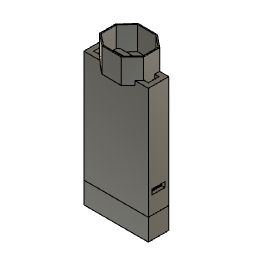
CasePCB v2 (Autodesk Fusion 360 design; units mm, degrees)
Autodesk Fusion 360 part; units mm, degrees
sketch "Schizzo1" plane through (0, 0, 0) normal (0, 0, 1) x (1, 0, 0)
  line L0 (-19.736, -1.3664) -> (-19.736, -16.3664)
  line L1 (19.7877, 0.2123) -> (19.7877, -14.7877)
  line L2 (-9.736, 9.5291) -> (8.264, 9.5291)
  line L3 (-19.736, -16.3664) -> (-8.7555, -25.0514)
  line L4 (19.7877, 0.2123) -> (8.264, 9.5291)
  line L5 (19.7877, -14.7877) -> (9.5787, -25.3157)
  line L6 (9.5787, -25.3157) -> (-8.7555, -25.0514)
  line L7 (-19.736, -1.3664) -> (-9.736, 9.5291)
  dimension "d1" = 15
  dimension "d2" = 15
  dimension "d3" = 18
  dimension "d5" = 18
  dimension "d6" = 18
  dimension "d10" = 14
  constraint vertical L0
  constraint vertical L1
  constraint horizontal L2
  measures "d1" distance of L0.start L0.end
  measures "d2" distance of L1.start L1.end
  measures "d3" distance of L2.start L2.end
  measures "d5" distance of L2.start L2.end
  measures "d6" distance of L2.start L2.end
  measures "d10" distance of L0.end L3.end
sketch "Schizzo2" plane through (0, 0, 0) normal (0, 0, 1) x (1, 0, 0)
extrude "Estrusione1" add sketch "Schizzo1" along normal blind 23 makes body 1
shell "Svuotamento1" thickness 1 removed faces 1 at (3.029, -13.6127, 23) on bodies 1
sketch "Schizzo3" plane through (0, 0, 0) normal (0, 0, -1) x (1, 0, 0)
  line L0 (-8.7555, 25.0514) -> (-19.736, 16.3664)
  line L1 (-19.736, 16.3664) -> (-19.736, 1.3664)
  line L2 (-19.736, 1.3664) -> (-9.736, -9.5291)
  line L3 (-9.736, -9.5291) -> (8.264, -9.5291)
  line L4 (8.264, -9.5291) -> (19.7877, -0.2123)
  line L5 (19.7877, -0.2123) -> (19.7877, 14.7877)
  line L6 (19.7877, 14.7877) -> (9.5787, 25.3157)
  line L7 (9.5787, 25.3157) -> (-8.7555, 25.0514)
  line L8 (-31.6305, 18.908) -> (28.3695, 18.908)
  line L9 (28.3695, 18.908) -> (28.3695, 0)
  line L10 (28.3695, 0) -> (-31.6305, 0)
  line L11 (-31.6305, 0) -> (-31.6305, 18.908)
  dimension "d48" = 60
  constraint horizontal L8
  constraint vertical L9
  constraint horizontal L10
  constraint vertical L11
  measures "d48" distance of L9 L11
extrude "Estrusione2" add sketch "Schizzo3" along normal blind 120 contours L0 L1 L2 L5 L6 L8 L10 | L0 L1 L2 L8 L10 L11 | L5 L6 L8 L9 L10 bodies 1
ref_plane "Piano di lavoro1" through (-1.6305, -9.454, -100) normal (0, 0, -1) x (-1, 0, 0)
split "Dividi1" by plane through (-1.6305, -9.454, -100) normal (0, 0, -1) bodies 1 makes body 2 at (8.3695, 0, -106.6667)
shell "Svuotamento2" thickness 3 removed faces 1 at (8.3695, -6.3027, -100) on bodies 1
shell "Svuotamento3" thickness 3 removed faces 1 at (8.3695, -6.3027, -100) on bodies 2
sketch "Schizzo4" plane through (0, 0, 0) normal (0, 0, 1) x (1, 0, 0)
  line L0 (-31.6305, -18.908) -> (-31.6305, 0)
  line L1 (-31.6305, 0) -> (28.3695, 0)
  line L2 (28.3695, 0) -> (28.3695, -18.908)
  line L3 (28.3695, -18.908) -> (-31.6305, -18.908)
  line L4 (-28.6305, -15.908) -> (25.3695, -15.908)
  line L5 (-28.6305, -3) -> (-28.6305, -15.908)
  line L6 (25.3695, -3) -> (-28.6305, -3)
  line L7 (25.3695, -15.908) -> (25.3695, -3)
  line L8 (23.8695, -14.408) -> (23.8695, -4.5)
  line L9 (23.8695, -4.5) -> (-27.1305, -4.5)
  line L10 (-27.1305, -4.5) -> (-27.1305, -14.408)
  line L11 (-27.1305, -14.408) -> (23.8695, -14.408)
  line L12 (29.8695, 1.5) -> (-33.1305, 1.5)
  line L13 (-33.1305, 1.5) -> (-33.1305, -20.408)
  line L14 (-33.1305, -20.408) -> (29.8695, -20.408)
  line L15 (29.8695, -20.408) -> (29.8695, 1.5)
  dimension "d22" = -1.5
  dimension "d23" = 4.5
extrude "Estrusione3" add sketch "Schizzo4" along normal blind 4 separate body contours L0 L1 L2 L3 | L4 L5 L6 L7 makes body 3
extrude "Estrusione4" add 1 faces at (-10.1305, -1.5, 0) along direction (0, 0, -1) blind 70 on bodies 3 bodies 3 1
extrude "Estrusione5" cut 1 faces at (-10.1305, -3.5, -70) along direction (0, 0, 1) blind 10 on bodies 3 bodies 3
sketch "Schizzo5" plane through (0, 0, -100) normal (0, 0, 1) x (-1, 0, 0)
  line L0 (-25.3695, 3) -> (-25.3695, 15.908)
  line L1 (-25.3695, 15.908) -> (28.6305, 15.908)
  line L2 (28.6305, 15.908) -> (28.6305, 3)
  line L3 (28.6305, 3) -> (-25.3695, 3)
  line L4 (31.6305, 0) -> (31.6305, 18.908)
  line L5 (31.6305, 18.908) -> (-28.3695, 18.908)
  line L6 (-28.3695, 18.908) -> (-28.3695, 0)
  line L7 (-28.3695, 0) -> (31.6305, 0)
  line L8 (-23.8695, 4.5) -> (-23.8695, 14.408)
  line L9 (-23.8695, 14.408) -> (27.1305, 14.408)
  line L10 (27.1305, 14.408) -> (27.1305, 4.5)
  line L11 (27.1305, 4.5) -> (-23.8695, 4.5)
  line L12 (-23.1825, 5.187) -> (-23.1825, 13.721)
  line L13 (-23.1825, 13.721) -> (26.4435, 13.721)
  line L14 (26.4435, 13.721) -> (26.4435, 5.187)
  line L15 (26.4435, 5.187) -> (-23.1825, 5.187)
  dimension "d31" = 1.5
  dimension "d32" = 2.187
extrude "Estrusione6" add sketch "Schizzo5" along normal blind 5 separate body contours L0 L1 L2 L3 | L8 L9 L10 L11 makes body 4
ref_plane "Piano di lavoro2" through (-1.6305, -9.454, -48) normal (0, 1, 0) x (-1, 0, 0)
sketch "Schizzo6" plane through (-0.5357, -9.454, -40) normal (0, 1, 0) x (1, 0, 0)
sketch "Schizzo7" plane through (-0.5357, -9.454, -40) normal (0, 1, 0) x (1, 0, 0)
  line L0 (-31.0949, 60) -> (28.9051, 60)
  line L1 (28.9051, 60) -> (28.9051, 80)
  line L2 (28.9051, 80) -> (-31.0949, 80)
  line L3 (-31.0949, 80) -> (-31.0949, 60)
  line L4 (25.9051, 60) -> (-28.0949, 60)
  line L5 (-28.0949, 60) -> (-28.0949, 55)
  line L6 (-28.0949, 55) -> (25.9051, 55)
  line L7 (25.9051, 55) -> (25.9051, 60)
  line L8 (20.1044, 55) -> (20.1044, 40)
  line L9 (20.1044, 40) -> (23.7181, 40)
  line L10 (23.7181, 40) -> (26.1861, 42.6476)
  line L11 (26.1861, 42.6476) -> (21.9112, 42.6476)
  line L12 (21.9112, 42.6476) -> (21.9112, 55)
  line L13 (21.9112, 55) -> (20.1044, 55)
  line L14 (20.1044, 55) -> (20.1044, 80)
  point P0 (23.7181, 55)
  point P1 (-25.9079, 55)
  dimension "d35" = 1.8069
  dimension "d36" = 15
  dimension "d37" = 2.6476
  dimension "d38" = 3.6138
  dimension "d39" = 42.989
  dimension "d40" = 25
  constraint coincident L6 L8.start
  constraint perpendicular L6 L8
  constraint perpendicular L8 L9
  constraint perpendicular L8 L11
  constraint coincident L6 L12.end
  constraint perpendicular L6 L12
  constraint coincident L2 L14.end
  constraint perpendicular L2 L14
  measures "d35" distance of P0 L12
  measures "d36" distance of L8.start L8.end
  measures "d37" vertical distance of L9.end L10.end
  measures "d38" distance of L8 L9.end
  measures "d39" angle of L1 L10
  measures "d40" distance of L8.start L14.end
extrude "Estrusione7" add sketch "Schizzo7" along normal mid plane 10 contours L0 L1 L2 L4 L14 | L0 L4 L6 L7 L13 L14 | L6 L8 L9 L10 L11 L12 L13 bodies 2 4
sketch "Schizzo8" plane through (28.3695, 0, 0) normal (1, 0, 0) x (0, 1, 0)
  line L0 (-18.908, 4) -> (-18.908, -100)
  line L1 (-18.908, -100) -> (0, -100)
  line L2 (0, -100) -> (0, 4)
  line L3 (-4.454, -80) -> (-14.454, -80)
  line L4 (-14.454, -80) -> (-14.454, -82.6476)
  line L5 (-14.454, -82.6476) -> (-4.454, -82.6476)
  line L6 (-4.454, -82.6476) -> (-4.454, -80)
  line L7 (-15.454, -79) -> (-15.454, -83.6476)
  line L8 (-15.454, -83.6476) -> (-3.454, -83.6476)
  line L9 (-3.454, -83.6476) -> (-3.454, -79)
  line L10 (-3.454, -79) -> (-15.454, -79)
  line L11 (0, 4) -> (-18.908, 4)
  dimension "d43" = 1
extrude "Estrusione8" cut sketch "Schizzo8" against normal through all contours L3 L4 L5 L6 | L7 L8 L9 L10 bodies 3
ref_plane "Piano di lavoro3" through (-1.6305, -9.454, -60) normal (-1, 0, 0) x (0, 1, 0)
mirror "Specchio1" about plane through (-1.6305, -9.454, -60) normal (-1, 0, 0) of "Estrusione7"
sketch "Schizzo9" plane through (0, 0, 0) normal (0, 1, 0) x (-1, 0, 0)
  line L0 (-28.3695, 4) -> (-28.3695, -100)
  line L1 (-28.3695, -100) -> (31.6305, -100)
  line L2 (31.6305, -100) -> (31.6305, 4)
  line L3 (18.4819, 0) -> (-19.7877, 0)
  line L4 (31.6305, 4) -> (18.4819, 4)
  line L5 (18.4819, 4) -> (18.4819, 0)
  line L6 (-19.7877, 0) -> (-19.7877, 4)
  line L7 (-19.7877, 4) -> (-28.3695, 4)
sketch "Schizzo10" plane through (28.3695, 0, 0) normal (1, 0, 0) x (0, 1, 0)
  line L0 (-3.454, -79) -> (-3.454, -83.6476)
  line L1 (-3.454, -83.6476) -> (-15.454, -83.6476)
  line L2 (-15.454, -83.6476) -> (-15.454, -79)
  line L3 (-15.454, -79) -> (-3.454, -79)
  line L4 (0, -100) -> (0, 4)
  line L5 (0, 4) -> (-18.908, 4)
  line L6 (-18.908, 4) -> (-18.908, -100)
  line L7 (-18.908, -100) -> (0, -100)
sketch "Schizzo11" plane through (-1.6305, 0, -48) normal (0, 1, 0) x (-1, 0, 0)
  circle A0 centre (-0.3, 16.2867) radius 4
  circle A1 centre (-0.3, 36.7357) radius 4
  dimension "d49" = 8
  dimension "d50" = 8
  measures "d49" diameter of A0
  measures "d50" diameter of A1
extrude "Estrusione9" cut sketch "Schizzo11" against normal blind 3 contours A0 bodies 3
extrude "Estrusione10" cut sketch "Schizzo11" against normal blind 6 contours A1 bodies 3
extrude "Estrusione11" cut sketch "Schizzo11" against normal blind 6 contours A0 bodies 3
equation "altezzapcb = 120 mm"
equation "d16 = altezzapcb"
equation "parete = 3 mm"
equation "d20 = parete"
equation "d21 = parete"
equation "d22 = -parete / 2"
equation "d23 = 1.5 mm + parete"
equation "incastro = 5 mm"
equation "d31 = parete / 2"
equation "d33 = incastro"
equation "largezzapcb = 60 mm"
equation "d48 = largezzapcb"
equation "d51 = -parete"
equation "d53 = -2 * parete"
equation "d55 = -2 * parete"
